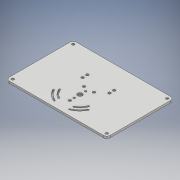
# Autodesk Inventor part: SheetPot
Saved by Autodesk Inventor 2018 (Build 220112000, 112)
## iProperties
Created: 2019-06-03
Part Number: SheetPot
Material: Generic
Document SubType Name: Modeling
Designer: aal_9
Density: 1 g/cm^3
Appearance: Default
Author: aal_9
Autodesk Inventor part; units mm, degrees
ref_plane "YZ Plane" through (0, 0, 0) normal (1, 0, 0) x (0, 1, 0)
ref_plane "XZ Plane" through (0, 0, 0) normal (0, 1, 0) x (-1, 0, 0)
ref_plane "XY Plane" through (0, 0, 0) normal (0, 0, 1) x (1, 0, 0)
sketch "Sketch1" plane through (0, 0, 0) normal (0, 0, 1) x (1, 0, 0)
  line L0 (-75, 65) -> (75, 65)
  line L1 (75, 65) -> (75, -35)
  line L2 (75, -35) -> (-75, -35)
  line L3 (-75, -35) -> (-75, 65)
  point P0 (0, 0)
  dimension "d0" = 150
  dimension "d1" = 100
  dimension "d26" = 75
  dimension "d27" = 65
  constraints: 8 end point, 2 parallel, 1 horizontal, 1 perpendicular
  measures "d0" distance of L0.start L0.end
  measures "d1" distance of L2.end L0.start
  measures "d26" distance from line of point (0, 0) L3
  measures "d27" distance from line of L0 point (0, 0)
extrude "Extrusion1" add sketch "Sketch1" along normal blind 3.175
sketch "Sketch2" plane through (0, 0, 3.175) normal (0, 0, 1) x (1, 0, 0)
  line L0 (75, 65) -> (-75, 65) projected
  line L1 (-75, 65) -> (-75, -35) projected
  line L2 (75, -35) -> (75, 65) projected
  line L3 (-75, -35) -> (75, -35) projected
  point P0 (0, 0)
  point P1 (-70, 60)
  point P2 (70, 60)
  point P3 (70, -30)
  point P4 (-70, -30)
  dimension "d4" = 5
  dimension "d5" = 5
  dimension "d6" = 5
  dimension "d7" = 5
  dimension "d8" = 5
  dimension "d9" = 5
  dimension "d10" = 5
  dimension "d11" = 5
  measures "d4" distance from line of L0 point (-70, 60)
  measures "d5" distance from line of L1 point (-70, 60)
  measures "d6" distance from line of L0 point (70, 60)
  measures "d7" distance from line of L2 point (70, 60)
  measures "d8" distance from line of L3 point (-70, -30)
  measures "d9" distance from line of L1 point (-70, -30)
  measures "d10" distance from line of L2 point (70, -30)
  measures "d11" distance from line of L3 point (70, -30)
hole "Hole1" at (-70, 60, 3.175) at (70, 60, 3.175) at (70, -30, 3.175) at (-70, -30, 3.175) direction (0, 0, -1) diameter 3 end through all countersink diameter 4 countersink angle 90
fillet "Fillet1" radius 5 4 edges at (-75, 65, 1.5875) (75, 65, 1.5875) (75, -35, 1.5875) (-75, -35, 1.5875)
sketch "Sketch4" plane through (0, 0, 0) normal (0, 0, -1) x (-1, 0, 0)
  circle A0 centre (0, 0) radius 3.5
  circle A1 centre (0, 8.5) radius 1.5
  circle A2 centre (0, -8.5) radius 1.5
  dimension "d35" = 7
  dimension "d36" = 8.5
  dimension "d37" = 8.5
  dimension "d38" = 3
  dimension "d39" = 3
  dimension "d40" = 0
  dimension "d41" = 0
  constraints: 3 centre point, 1 coincident
  measures "d35" diameter of A0
  measures "d36" distance of A0.centre A1.centre
  measures "d37" distance of A0.centre A2.centre
  measures "d38" diameter of A2
  measures "d39" diameter of A1
  measures "d40" horizontal distance of point (0, 0) A1.centre
  measures "d41" horizontal distance of point (0, 0) A2.centre
extrude "Extrusion3" cut sketch "Sketch4" against normal up to next
sketch "Sketch5" plane through (0, 0, 0) normal (0, 0, -1) x (-1, 0, 0)
  line L0 (5.9999, -30) -> (5.9999, 8.0565) construction
  line L1 (11.1182, -28.5024) -> (4.5396, 8.8062) construction
  line L2 (15.8986, -26.1386) -> (3.2654, 8.571) construction
  line L3 (20.1961, -22.9808) -> (2.6287, 7.447) construction
  line L4 (23.8798, -19.1247) -> (2.1665, 6.7525) construction
  line L5 (-70, -35) -> (70, -35) projected
  line L6 (75, -30) -> (75, 60) projected
  line L7 (10.5712, -25.4002) -> (13.7361, -24.8422)
  line L8 (14.8213, -23.1786) -> (18.4034, -21.8748) construction
  line L9 (18.6211, -20.2528) -> (20.9099, -18.9314) construction
  line L10 (21.855, -16.7116) -> (23.791, -15.0872) construction
  arc A0 (11.1499, -20.35) -> (17.4375, -15.3092) centre (0.0019, -0.0027) ccw construction
  arc A1 (17.4375, -15.3092) -> (21.6221, -8.422) centre (0.0014, -0.0005) ccw construction
  arc A2 (11.1499, -26.85) -> (19.6607, -21.4172) centre (0.0018, -0.0031) ccw construction
  arc A3 (19.6607, -21.4172) -> (25.8002, -13.4013) centre (0.0012, -0.0006) ccw construction
  arc A4 (11.1499, -20.35) -> (21.6221, -8.422) centre (-0.0011, 0.001) ccw construction
  arc A5 (11.6424, -21.2489) -> (22.5772, -8.794) centre (-0.0011, 0.001) ccw
  arc A6 (10.6574, -19.4511) -> (20.667, -8.05) centre (-0.0011, 0.001) ccw
  arc A7 (10.6574, -19.4511) -> (11.6424, -21.2489) centre (11.1499, -20.35) ccw
  arc A8 (22.5772, -8.794) -> (20.667, -8.05) centre (21.6221, -8.422) ccw
  arc A9 (11.1499, -26.85) -> (25.8002, -13.4013) centre (-0.0009, 0.001) ccw construction
  arc A10 (11.543, -27.7966) -> (26.7098, -13.8738) centre (-0.0009, 0.001) ccw
  arc A11 (10.7568, -25.9034) -> (24.8906, -12.9288) centre (-0.0009, 0.001) ccw
  arc A12 (10.7568, -25.9034) -> (11.543, -27.7966) centre (11.1499, -26.85) ccw
  arc A13 (26.7098, -13.8738) -> (24.8906, -12.9288) centre (25.8002, -13.4013) ccw
  line L11 (0, -12.0487) -> (0, -35) construction
  arc A14 (-22.5772, -8.794) -> (-11.6424, -21.2489) centre (0.0011, 0.001) ccw
  arc A15 (-20.667, -8.05) -> (-10.6574, -19.4511) centre (0.0011, 0.001) ccw
  arc A16 (-11.6424, -21.2489) -> (-10.6574, -19.4511) centre (-11.1499, -20.35) ccw
  arc A17 (-20.667, -8.05) -> (-22.5772, -8.794) centre (-21.6221, -8.422) ccw
  arc A18 (-26.7098, -13.8738) -> (-11.543, -27.7966) centre (0.0009, 0.001) ccw
  arc A19 (-24.8906, -12.9288) -> (-10.7568, -25.9034) centre (0.0009, 0.001) ccw
  arc A20 (-11.543, -27.7966) -> (-10.7568, -25.9034) centre (-11.1499, -26.85) ccw
  arc A21 (-24.8906, -12.9288) -> (-26.7098, -13.8738) centre (-25.8002, -13.4013) ccw
  point P0 (0, 0)
  point P1 (15.643, -24.5059)
  point P2 (14.5143, -18.1047)
  point P3 (23.0811, -17.6778)
  point P4 (19.8311, -12.0486)
  dimension "d48" = 5.15
  dimension "d50" = 3.15
  dimension "d51" = 6.5
  dimension "d52" = 5.15
  dimension "d53" = 5.15
  dimension "d54" = 3.15
  dimension "d55" = 0
  dimension "d56" = 5.15
  dimension "d57" = 6.5
  dimension "d58" = 5.15
  dimension "d59" = 5.15
  dimension "d60" = 3.15
  dimension "d61" = 0
  dimension "d62" = 6.5
  dimension "d63" = 5.15
  dimension "d64" = 5.15
  dimension "d65" = 3.15
  dimension "d66" = 0
  dimension "d67" = 6.5
  dimension "d68" = 5.15
  dimension "d69" = 5.15
  dimension "d70" = 3.15
  dimension "d71" = 0
  dimension "d72" = 6.5
  dimension "d73" = 2.05
  dimension "d74" = 2.05
  dimension "d75" = 22.9513
  constraints: 50 point on circle, 22 centre point, 20 end point, 14 symmetric about line, 8 tangent, 4 perpendicular, 4 point on line, 2 vertical, 1 midpoint, 23 other
  measures "d48" horizontal distance of A2.start L0.start
  measures "d50" vertical distance of L0.start A2.start
  measures "d51" distance of A2.start A0.start
  measures "d52" horizontal distance of L0.start A0.start
  measures "d53" distance from line of point (15.643, -24.506) L1
  measures "d54" distance from line of L1.start L7
  measures "d55" distance from line of L7 point (15.643, -24.506)
  measures "d56" distance from line of L1 point (14.514, -18.105)
  measures "d57" distance from line of L7 point (14.514, -18.105)
  measures "d58" distance from line of A2.end L2
  measures "d59" distance from line of L2 A0.end
  measures "d60" distance from line of L2.start L8
  measures "d61" distance from line of L8 A2.end
  measures "d62" distance from line of L8 A0.end
  measures "d63" distance from line of point (23.081, -17.678) L3
  measures "d64" distance from line of L3 point (19.831, -12.049)
  measures "d65" distance from line of L3.start L9
  measures "d66" distance from line of point (23.081, -17.678) L9
  measures "d67" distance from line of L9 point (19.831, -12.049)
  measures "d68" distance from line of L4 A3.end
  measures "d69" distance from line of L4 A1.end
  measures "d70" distance from line of L4.start L10
  measures "d71" distance from line of A3.end L10
  measures "d72" distance from line of L10 A1.end
  measures "d73" diameter of A8
  measures "d74" diameter of A13
  measures "d75" distance of L11.start L11.end
extrude "Extrusion4" cut sketch "Sketch5" against normal through all
sketch "Sketch8" plane through (0, 0, 3.175) normal (0, 0, 1) x (1, 0, 0)
  point P0 (0, 0)
  point P1 (-7.5, 13.5)
  point P2 (7.5, 13.5)
  point P3 (0, -15)
  dimension "d78" = 7.5
  dimension "d79" = 15
  dimension "d80" = 13.5
  dimension "d81" = 13.5
  dimension "d82" = 15
  dimension "d83" = 0
  measures "d78" horizontal distance of point (0, 0) point (-7.5, 13.5)
  measures "d79" distance of point (-7.5, 13.5) point (7.5, 13.5)
  measures "d80" vertical distance of point (0, 0) point (-7.5, 13.5)
  measures "d81" vertical distance of point (0, 0) point (7.5, 13.5)
  measures "d82" distance of point (0, 0) point (0, -15)
  measures "d83" horizontal distance of point (0, 0) point (0, -15)
hole "Hole2" at (-7.5, 13.5, 3.175) at (7.5, 13.5, 3.175) at (0, -15, 3.175) direction (0, 0, -1) diameter 3 end through all countersink diameter 4 countersink angle 90
sketch "Sketch9" plane through (0, 0, 3.175) normal (0, 0, 1) x (1, 0, 0)
  line L0 (70, 65) -> (-70, 65) projected
  line L1 (-75, 60) -> (-75, -30) projected
  point P0 (0, 0)
  point P1 (-20, 31)
  point P2 (-20, 24)
  point P3 (20, 24)
  point P4 (20, 31)
  dimension "d91" = 40
  dimension "d92" = 34
  dimension "d93" = 7
  dimension "d94" = 7
  dimension "d95" = 34
  dimension "d96" = 55
  dimension "d97" = 55
  dimension "d98" = 40
  measures "d91" distance of point (20, 31) point (-20, 31)
  measures "d92" distance from line of L0 point (-20, 31)
  measures "d93" distance of point (-20, 31) point (-20, 24)
  measures "d94" distance of point (20, 31) point (20, 24)
  measures "d95" distance from line of L0 point (20, 31)
  measures "d96" distance from line of L1 point (-20, 31)
  measures "d97" distance from line of point (-20, 24) L1
  measures "d98" distance of point (-20, 24) point (20, 24)
hole "Hole3" at (-20, 31, 3.175) at (-20, 24, 3.175) at (20, 24, 3.175) at (20, 31, 3.175) direction (0, 0, -1) diameter 3 end through all countersink diameter 4 countersink angle 90
equation "\"d78\" = 0.5 * d79"
body "Solid1"
